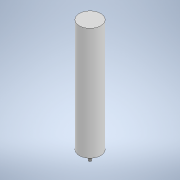
# Autodesk Inventor part: Boquilla0.25
Saved by Autodesk Inventor 2022 (Build 260153000, 153)
## iProperties
Created: 2022-04-01
Part Number: Boquilla0.25
Material: Genérico
Document SubType Name: Modeling
Designer: anuar
Density: 1 g/cm^3
Appearance: Valor por defecto
Author: anuar
Autodesk Inventor part; units mm, degrees
ref_plane "YZ Plane" through (0, 0, 0) normal (1, 0, 0) x (0, 1, 0)
ref_plane "XZ Plane" through (0, 0, 0) normal (0, 1, 0) x (-1, 0, 0)
ref_plane "XY Plane" through (0, 0, 0) normal (0, 0, 1) x (1, 0, 0)
sketch "Boceto1" plane through (0, 0, 0) normal (0, 0, 1) x (1, 0, 0)
  line L0 (0.125, 0) -> (0.125, 0.38)
  line L1 (0.125, 0.38) -> (1, 0.8852)
  line L2 (1, 0.8852) -> (1, 11.3952)
  line L3 (-0.198, 0) -> (1.188, 0) projected
  line L4 (1, 11.3952) -> (0, 11.3952)
  line L5 (0, 0) -> (0.125, 0)
  line L6 (0, 11.3952) -> (0, 0)
  dimension "d1" = 0.125
  dimension "d2" = 0.38
  dimension "d4" = 10.51
  dimension "d8" = 60
  dimension "d9" = 1
  constraints: 12 end point, 1 collinear, 1 parallel, 1 point on line
  measures "d1" distance from line of L5.start L0
  measures "d2" distance of L0.start L0.end
  measures "d4" distance of L1.end L2.end
  measures "d8" angle of L6 L1
  measures "d9" distance between parallel lines of L6 L2
revolve "Revolución1" add sketch "Boceto1" angle 360 about axis through (0, 11.3952, 0) along (0, -1, 0)
equation "\"d1\" = 0.5 * Dc"
equation "\"d2\" = Lc"
equation "\"d4\" = Ln"
equation "\"d8\" = alfa"
equation "\"d9\" = 0.5 * Do"
equation "\"Dc\" = 0.25"
equation "\"Lc\" = 0.38"
equation "\"Ln\" = 10.51"
equation "\"Do\" = 2"
equation "\"alfa\" = 60deg"
